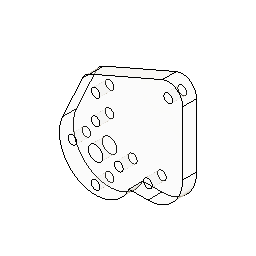
AssemblyThrowerMotor v5 (Autodesk Fusion 360 archive; units mm, degrees)
design "ThrowerMotorJunction"
Autodesk Fusion 360 part; units mm, degrees
sketch "Sketch1" plane through (0, 0, 0) normal (0, 1, 0) x (1, 0, 0)
  circle A0 centre (0, 0) radius 8 construction
  circle A1 centre (0, 0) radius 9.5 construction
  circle A2 centre (0, 0) radius 14 construction
  circle A3 centre (0, 0) radius 18 construction
  line L0 (0, 0) -> (0, -18) construction
  line L1 (0, 0) -> (0, 52) construction
  line L2 (0, 0) -> (18, 0) construction
  line L3 (0, 0) -> (-18, 0) construction
  circle A4 centre (0, 0) radius 48 construction
  circle A5 centre (0, 0) radius 58 construction
  line L4 (0, 47) -> (-33.9853, 47) construction
  circle A6 centre (0, -9.5) radius 1.5
  circle A7 centre (-8, 0) radius 1.5
  circle A8 centre (8, 0) radius 1.5
  circle A9 centre (0, 9.5) radius 1.5
  circle A10 centre (18, 0) radius 1.5
  circle A11 centre (0, -18) radius 1.5
  line L5 (-50.3158, -28.85) -> (25, -28.85) construction
  circle A12 centre (25, -28.85) radius 1.5
  line L6 (-11.3632, -5.2083) -> (-4.1251, -21)
  line L7 (11.4564, 5) -> (18, 5)
  line L8 (30, -7) -> (30, -28.85)
  arc A13 (12.5, 0) -> (11.4564, 5) centre (0, 0) ccw construction
  arc A14 (11.4564, 5) -> (-11.3632, -5.2083) centre (0, 0) ccw
  arc A15 (0, -12.5) -> (12.5, 0) centre (0, 0) ccw construction
  arc A16 (-11.3632, -5.2083) -> (0, -12.5) centre (0, 0) ccw construction
  circle A17 centre (0, 0) radius 2.5
  arc A18 (30, -28.85) -> (23.0094, -33.4367) centre (25, -28.85) ccw construction
  arc A19 (23.0094, -33.4367) -> (30, -28.85) centre (25, -28.85) ccw
  line L9 (-1.9906, -22.5867) -> (23.0094, -33.4367)
  arc A20 (-1.9906, -22.5867) -> (-4.5453, -20.0833) centre (0, -18) ccw construction
  arc A21 (-4.5453, -20.0833) -> (-1.9906, -22.5867) centre (0, -18) ccw
  arc A22 (18, 5) -> (30, -7) centre (18, -7) ccw construction
  arc A23 (30, -7) -> (18, 5) centre (18, -7) ccw
  point P0 (0, 14)
  point P1 (0, 47)
  point P2 (-47.869, 32.75)
  point P3 (-42.1187, 39.875)
  point P4 (-50.8212, 27.95)
  point P5 (-55.4373, -17.05)
  point P6 (-53.7269, -21.85)
  point P7 (-50.3158, -28.85)
  point P8 (0, 9.5)
  point P9 (8, 0)
  point P10 (0, 12.5)
  dimension "d19" = 16
  dimension "d20" = 19
  dimension "d21" = 28
  dimension "d22" = 36
  dimension "d23" = 38
  dimension "d24" = 96
  dimension "d25" = 116
  dimension "d26" = 5
  dimension "d27" = 19.25
  dimension "d28" = 4.8
  dimension "d29" = 7.125
  dimension "d30" = 45
  dimension "d31" = 4.8
  dimension "d32" = 7
  dimension "d33" = 3
  dimension "d34" = 3
  dimension "d35" = 3
  dimension "d36" = 3
  dimension "d37" = 3
  dimension "d38" = 3
  dimension "d39" = 25
  dimension "d40" = 3
  dimension "d41" = 3
  dimension "d44" = 5
  dimension "d45" = 5
  dimension "d48" = 5
  dimension "d49" = 3
  dimension "d50" = 5
  dimension "d51" = 12
  constraint coincident A0.centre A1.centre
  constraint concentric A0 A2
  constraint concentric A1 A3
  constraint coincident A3 L0.end
  constraint vertical L0
  constraint parallel L0 L1
  constraint coincident A3 L2.end
  constraint horizontal L2
  constraint coincident A3 L3.end
  constraint parallel L2 L3
  constraint coincident A2 P0
  constraint coincident L1 P0
  constraint concentric A0 A4
  constraint concentric A3 A5
  constraint coincident L1 P1
  constraint coincident P1 L4.start
  constraint coincident A5 L4.end
  constraint perpendicular L1 L4
  constraint coincident A5 P2
  constraint coincident A5 P3
  constraint coincident A5 P4
  constraint coincident A5 P5
  constraint coincident A5 P6
  constraint coincident A5 P7
  constraint coincident A1 A6.centre
  constraint coincident L0 A6.centre
  constraint coincident A1 P8
  constraint coincident L1 P8
  constraint coincident A0 A7.centre
  constraint coincident L3 A7.centre
  constraint coincident A0 P9
  constraint coincident L2 P9
  constraint coincident P9 A8.centre
  constraint coincident P8 A9.centre
  constraint coincident L2.end A10.centre
  constraint coincident L0.end A11.centre
  constraint coincident P7 L5.start
  constraint horizontal L5
  constraint coincident L5.end A12.centre
  constraint concentric A3 A14
  constraint coincident L1 P10
  constraint coincident P10 A14
  constraint tangent L6 A14
  constraint horizontal L7
  constraint perpendicular L7 L8
  constraint coincident L2 A13.start
  constraint concentric A13 A14
  constraint coincident L0 A15.start
  constraint concentric A14 A15
  constraint concentric A14 A16
  constraint concentric A5 A17
  constraint concentric A12 A18
  constraint tangent L8 A18
  constraint concentric A18 A19
  constraint concentric A11 A20
  constraint tangent L6 A20
  constraint tangent A18 L9
  constraint tangent L9 A20
  constraint coincident L6 A20.end
  constraint concentric A20 A21
  constraint tangent L8 A22
  constraint tangent L7 A22
  constraint concentric A22 A23
  measures "d19" diameter of A0
  measures "d20" diameter of A1
  measures "d21" diameter of A2
  measures "d22" diameter of A3
  measures "d23" distance of L1.end P0
  measures "d24" diameter of A4
  measures "d25" diameter of A5
  measures "d26" distance of L1.end P1
  measures "d27" vertical distance of L1.end P2
  measures "d28" vertical distance of P2 P4
  measures "d29" vertical distance of P2 P3
  measures "d30" vertical distance of P4 P5
  measures "d31" vertical distance of P5 P6
  measures "d32" vertical distance of P6 P7
  measures "d33" diameter of A6
  measures "d34" diameter of A7
  measures "d35" diameter of A8
  measures "d36" diameter of A9
  measures "d37" diameter of A10
  measures "d38" diameter of A11
  measures "d39" horizontal distance of L0.end L5.end
  measures "d40" diameter of A12
  measures "d41" distance of P8 P10
  measures "d44" distance of L2.end L7
  measures "d45" distance of L5.end L8
  measures "d48" diameter of A17
  measures "d49" vertical distance of L6.end L0.end
  measures "d50" radius of A20
  measures "d51" distance of L8 A22.centre
extrude "Extrude1" add sketch "Sketch1" along normal blind 4.8

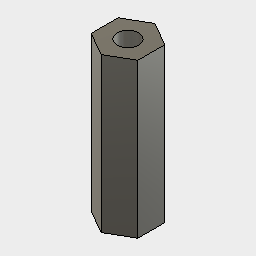
design "Spacer M3x18"
Autodesk Fusion 360 part; units mm, degrees
sketch "Sketch1" plane through (0, 0, 0) normal (0, 1, 0) x (1, 0, 0)
  line L0 (2.725, 1.5733) -> (0, 3.1466)
  line L1 (0, 3.1466) -> (-2.725, 1.5733)
  line L2 (-2.725, 1.5733) -> (-2.725, -1.5733)
  line L3 (-2.725, -1.5733) -> (0, -3.1466)
  line L4 (0, -3.1466) -> (2.725, -1.5733)
  line L5 (2.725, -1.5733) -> (2.725, 1.5733)
  circle A0 centre (0, 0) radius 1.25
  dimension "d1" = 2.5
  measures "d1" diameter of A0
extrude "Extrude1" add sketch "Sketch1" along normal blind 18
